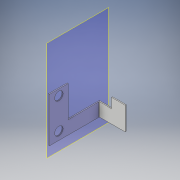
# Autodesk Inventor part: Fixação com Tanque - DIN
Saved by Autodesk Inventor 2019 (Build 230136000, 136)
## iProperties
Created: 2015-09-14
Part Number: Fixação com Tanque - DIN
Material: Genérico
Document SubType Name: Modeling
Designer: BAJA UEA
Density: 1 g/cm^3
Appearance: Padrão
Mass: 4352.78 g
Surface Area: 3520.72 cm^2
Volume: 4352.78 cm^3
Author: BAJA UEA
Autodesk Inventor part; units mm, degrees
ref_plane "YZ Plane" through (0, 0, 0) normal (1, 0, 0) x (0, 1, 0)
ref_plane "XZ Plane" through (0, 0, 0) normal (0, 1, 0) x (-1, 0, 0)
ref_plane "XY Plane" through (0, 0, 0) normal (0, 0, 1) x (1, 0, 0)
ref_plane "Plano de trabalho2" through (-1094.0332, 123.1084, -225.312) normal (0, 1, 0) x (1, 0, 0)
sketch "Esboço10" plane through (-1094.0332, 123.1084, -225.312) normal (0, 1, 0) x (1, 0, 0)
  line L0 (115.9279, 81.534) -> (115.9279, -34.0424)
  line L1 (115.9279, 81.534) -> (115.9279, 81.534)
  line L2 (115.9279, 81.534) -> (115.9279, -5.1435)
  circle A0 centre (115.9279, -5.1435) radius 8.001
  line L3 (115.9279, 81.534) -> (115.9279, 52.6415)
  circle A1 centre (115.9279, 52.6415) radius 8.001
  line L4 (98.0571, -16.7405) -> (133.6171, -16.7405)
  line L5 (133.6171, -16.7405) -> (133.6171, 68.072)
  line L6 (133.6171, 68.072) -> (98.0571, 68.072)
  line L7 (98.0571, 68.072) -> (98.0571, -16.7405)
  line L8 (133.6171, 68.072) -> (194.8819, 68.072)
  line L9 (133.6171, 68.072) -> (194.8819, 68.072) construction
  line L10 (194.8819, 68.072) -> (194.8819, 42.672)
  line L11 (194.8819, 42.672) -> (133.6171, 42.672)
  circle A2 centre (194.8891, 22.0646) radius 12.7
  line L12 (133.6171, 68.072) -> (133.6171, 42.672)
  line L13 (133.6171, 68.072) -> (194.8819, 68.072)
  line L14 (194.8819, 68.072) -> (194.8819, 42.672)
  line L15 (194.8819, 42.672) -> (133.6171, 42.672)
  line L16 (133.6171, 42.672) -> (133.6171, 68.072)
  point P0 (1094.0332, -225.312)
  dimension "d30" = 0
  dimension "d34" = 86.6775
  dimension "d35" = 16.002
  dimension "d36" = 28.8925
  dimension "d37" = 16.002
  dimension "d38" = 35.56
  dimension "d41" = 61.2648
  dimension "d42" = 0
  dimension "d43" = 25.4
  dimension "d44" = 25.4
  constraints: 34 end point, 4 parallel, 4 perpendicular, 4 point on line, 3 centre point, 3 horizontal, 2 coincident, 2 collinear, 1 vertical
  measures "d30" distance of L0.start L1.end
  measures "d34" distance of L0.start L2.end
  measures "d35" diameter of A0
  measures "d36" distance of L0.start L3.end
  measures "d37" diameter of A1
  measures "d38" distance of L6.end L5.end
  measures "d41" distance of L5.end L8.end
  measures "d42" distance between parallel lines of L8 L9
  measures "d43" distance of L9.end L10.end
  measures "d44" diameter of A2
extrude "Extrusão9" add sketch "Esboço10" along normal blind 2 contours L6 L5 L4 L0 A0 A1 | L0 A1 A0 L4 L7 L6 | L8 L10 L11 L5
sketch "Esboço11" plane through (-899.1512, 123.1084, -267.984) normal (1, 0, 0) x (0, 0, -1)
  line L0 (0, 2) -> (25.4, 2) projected
  line L1 (25.4, 2) -> (0, 2)
  line L2 (0, 2) -> (0, -48.8)
  line L3 (0, -48.8) -> (25.4, -48.8)
  line L4 (25.4, -48.8) -> (25.4, 2)
  line L5 (0, -48.8) -> (-18.5597, -48.8)
  line L6 (-18.5597, -48.8) -> (-18.5597, -23.4)
  line L7 (-18.5597, -23.4) -> (0, -23.4)
  line L8 (0, -23.4) -> (0, -48.8)
  point P0 (-267.984, -123.1084)
  dimension "d45" = 25.4
  dimension "d46" = 50.8
  dimension "d48" = 25.4
  constraints: 16 end point, 4 parallel, 2 horizontal, 2 perpendicular
  measures "d45" distance of L3.end L2.end
  measures "d46" distance of L2.end L1.end
  measures "d48" distance of L5.end L6.end
extrude "Extrusão10" add sketch "Esboço11" against normal blind 2
fillet "Arredondamento1" radius 1 1 edges at (-899.1512, 125.1084, -280.684)
fillet "Arredondamento2" radius 1 1 edges at (-901.1512, 123.1084, -280.684)
thread "Rosca1" size "11/16-12 UN" class "2B" standard "ANSI Unified Screw Threads" full length
thread "Rosca2" size "11/16-12 UN" class "2B" standard "ANSI Unified Screw Threads" full length
body "Solid1"
